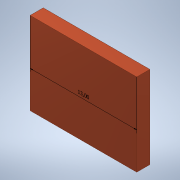
# Autodesk Inventor part: Placa Cobre
Saved by Autodesk Inventor 2020.3 (Build 243373000, 373)
## iProperties
Created: 2020-06-16
Part Number: Placa Cobre
Material: Cobre
Document SubType Name: Modeling
Designer: javic
Mass: 1.87068 g
Surface Area: 3.35352 cm^2
Volume: 0.209248 cm^3
Density: 8.94 g/cm^3
Appearance: Cobre - Satinado
Author: javic
Autodesk Inventor part; units mm, degrees
ref_plane "YZ Plane" through (0, 0, 0) normal (1, 0, 0) x (0, 1, 0)
ref_plane "XZ Plane" through (0, 0, 0) normal (0, 1, 0) x (-1, 0, 0)
ref_plane "XY Plane" through (0, 0, 0) normal (0, 0, 1) x (1, 0, 0)
sketch "Boceto1" plane through (0, 0, 0) normal (0, 1, 0) x (-1, 0, 0)
  line L0 (0, 0) -> (13, 0)
  line L1 (13, 0) -> (13, -1.6)
  line L2 (13, -1.6) -> (0, -1.6)
  line L3 (0, -1.6) -> (0, 0)
  dimension "d0" = 13
  dimension "d1" = 1.6
  constraints: 8 end point, 2 parallel, 1 horizontal, 1 perpendicular
  measures "d0" distance of L1.end L2.end
  measures "d1" distance of L0.end L1.end
extrude "Extrusión1" add sketch "Boceto1" along normal blind 10.06
